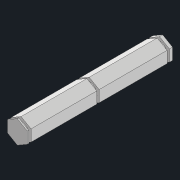
# Autodesk Inventor part: Drive Shaft
Saved by Autodesk Inventor 2022 (Build 260153000, 153)
## iProperties
Created: 2022-09-06
Part Number: Drive Shaft
Material: Generic
Document SubType Name: Modeling
Designer: robpl
Density: 1 g/cm^3
Appearance: Default
Author: robpl
Autodesk Inventor part; units mm, degrees
ref_plane "YZ Plane" through (0, 0, 0) normal (1, 0, 0) x (0, 1, 0)
ref_plane "XZ Plane" through (0, 0, 0) normal (0, 1, 0) x (-1, 0, 0)
ref_plane "XY Plane" through (0, 0, 0) normal (0, 0, 1) x (1, 0, 0)
sketch "Sketch1" plane through (0, 0, 0) normal (0, 0, 1) x (1, 0, 0)
  line L0 (6.35, -3.6662) -> (0, -7.3323)
  line L1 (0, -7.3323) -> (-6.35, -3.6662)
  line L2 (-6.35, -3.6662) -> (-6.35, 3.6662)
  line L3 (-6.35, 3.6662) -> (0, 7.3323)
  line L4 (0, 7.3323) -> (6.35, 3.6662)
  line L5 (6.35, 3.6662) -> (6.35, -3.6662)
  point P0 (0, 0)
  point P1 (0, 0)
  dimension "d0" = 12.7
  constraints: 12 end point, 1 coincident, 1 vertical, 13 other
  measures "d0" distance between parallel lines of L1 L4
extrude "Extrusion1" add sketch "Sketch1" along normal blind 94
sketch "Sketch2" plane through (0, 0, 0) normal (1, 0, 0) x (0, 1, 0)
  line L0 (15, 2) -> (5, 2)
  line L1 (5, 2) -> (5, 3.5)
  line L2 (5, 3.5) -> (15, 3.5)
  line L3 (15, 3.5) -> (15, 2)
  line L4 (3.6662, 0) -> (7.3323, 0) projected
  line L5 (0, -18.42) -> (0, 110.52) projected
  line L6 (15, 92.5) -> (5, 92.5)
  line L7 (5, 92.5) -> (5, 91)
  line L8 (5, 91) -> (15, 91)
  line L9 (15, 91) -> (15, 92.5)
  line L10 (15, 48.5) -> (5, 48.5)
  line L11 (5, 48.5) -> (5, 47)
  line L12 (5, 47) -> (15, 47)
  line L13 (15, 47) -> (15, 48.5)
  point P0 (0, 0)
  point P1 (0, 0)
  point P2 (15, 2.75)
  point P3 (15, 47.75)
  dimension "d3" = 1.5
  dimension "d4" = 2
  dimension "d5" = 10
  dimension "d6" = 5
  dimension "d8" = 91
  dimension "d9" = 47
  constraints: 24 end point, 6 parallel, 4 equal length, 3 horizontal, 3 perpendicular, 2 midpoint, 2 vertical alignment, 1 coincident
  measures "d3" distance of L2.end L0.start
  measures "d4" distance between parallel lines of L4 L0
  measures "d5" distance of L0.start L0.end
  measures "d6" distance from line of point (0, 0) L1
  measures "d8" distance between parallel lines of L8 L4
  measures "d9" distance between parallel lines of L4 L12
revolve "Revolution1" cut sketch "Sketch2" angle 360 about axis through (0, 0, -10) along (0, 0, 1)
body "Solid1"
